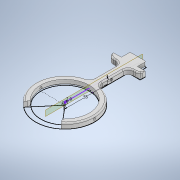
# Autodesk Inventor part: deadbolt enclosure reinforcer from doorknob
Saved by Autodesk Inventor 2022 (Build 260153000, 153)
## iProperties
Created: 2022-04-07
Part Number: deadbolt enclosure reinforcer from doorknob
Material: Generic
Document SubType Name: Modeling
Designer: a-dubs
Density: 1 g/cm^3
Appearance: Default
Author: a-dubs
Autodesk Inventor part; units mm, degrees
ref_plane "YZ Plane" through (0, 0, 0) normal (1, 0, 0) x (0, 1, 0)
ref_plane "XZ Plane" through (0, 0, 0) normal (0, 1, 0) x (-1, 0, 0)
ref_plane "XY Plane" through (0, 0, 0) normal (0, 0, 1) x (1, 0, 0)
sketch "Sketch1" plane through (0, 0, 0) normal (0, 1, 0) x (-1, 0, 0)
  circle A0 centre (0, 0) radius 30.5
  line L0 (0, -30.5) -> (0, -81)
  line L1 (0, -81) -> (0, -92)
  line L2 (0, -92) -> (-10.1, -92)
  line L3 (-10.1, -92) -> (-10.1, -81)
  line L4 (-10.1, -81) -> (0, -81)
  line L5 (-3.0031, -30.5) -> (-3.0031, -30.3518)
  line L6 (-3.0031, -30.5) -> (-3.0031, -81)
  line L7 (-10.1, -81) -> (-10.1, -74.6)
  line L8 (-10.1, -74.6) -> (-3.0031, -74.6)
  line L9 (0, -30.5) -> (0, -36.9)
  circle A1 centre (0, 0) radius 36.9
  line L10 (0, 0) -> (23.7189, 28.267)
  line L11 (0, 0) -> (36.9, 0) construction
  line L12 (0, 0) -> (-23.7189, 28.267)
  line L13 (0, 0) -> (36.9, 0) construction
  line L14 (-10.1, -81) -> (-19.7, -81)
  line L15 (-19.7, -81) -> (-19.7, -74.6)
  line L16 (-19.7, -74.6) -> (-10.1, -74.6)
  line L17 (0, -30.5) -> (-4.8, -30.5)
  line L18 (-4.8, -30.5) -> (-4.8, -30.1199)
  line L19 (-4.8, -30.5) -> (-4.8, -81)
  point P0 (-19.605, 23.3644)
  point P1 (-3.0031, -36.7776)
  point P2 (19.605, 23.3644)
  point P3 (-4.8, -36.5865)
  point P4 (-4.8, -74.6)
  dimension "d0" = 61
  dimension "d1" = 50.5
  dimension "d2" = 11
  dimension "d4" = 10.1
  dimension "d9" = 6.4
  dimension "d10" = 6.4
  dimension "d11" = 50
  dimension "d12" = 130
  dimension "d15" = 9.6
  dimension "d36" = 4.8
  constraints: 40 end point, 6 point on circle, 6 point on line, 5 horizontal, 5 perpendicular, 5 vertical, 2 centre point, 2 coincident, 2 equal length, 1 tangent
  measures "d0" diameter of A0
  measures "d1" distance of L0.start L0.end
  measures "d2" distance of L0.end L1.end
  measures "d4" distance of L1.end L2.end
  measures "d9" distance of L3.end L7.end
  measures "d10" distance of L0.start L9.end
  measures "d11" angle of L11 L10
  measures "d12" angle of L13 L12
  measures "d15" distance of L3.end L14.end
  measures "d36" distance of L0.start L17.end
extrude "Extrusion1" add sketch "Sketch1" along normal blind 6.4 contours L18 L19 A1 L12 A0 | A0 L5 L17 L18 | A0 L17 L5 | L17 L6 A1 L19 | L0 A1 L6 L17 | A1 L6 L8 L19 | L0 L4 L6 A1 | L19 L4 L7 L8 | L8 L6 L4 L19 | L1 L2 L3 L4 | L7 L14 L15 L16
fillet "Fillet1" radius 6.4 1 edges at (4.8, 3.2, -74.6)
chamfer "Chamfer1" distance 3.2 angle 45 1 edges at (19.7, 3.2, -74.6)
fillet "Fillet2" radius 6.4 1 edges at (16.5, 3.2, -74.6)
fillet "Fillet3" radius 6.4 1 edges at (4.8, 3.2, -36.5865)
ref_plane "Work Plane1" through (0, 3.2, -92) normal (-1, 0, 0) x (0, 0, 1)
fillet "Fillet4" radius 1.6 6 edges at (6.1229, 6.4, -37.9299) (36.0247, 6.4, -7.9896) (16.2982, 6.4, -75.0872) (19.0373, 6.4, -77.1373) (6.6745, 6.4, -72.7255) (10.1, 3.2, -92)
mirror "Mirror1" about plane through (0, 3.2, -92) normal (-1, 0, 0) of "Extrusion1", "Fillet3", "Fillet4", "Fillet2", "Chamfer1", "Fillet1"
chamfer "Chamfer2" distance 1.6 angle 45 5 edges at (4.25, 0, -92) (-9.6314, 0, -91.5314) (-10.1, 0, -85.7) (9.6314, 0, -91.5314) (10.1, 0, -85.7)
chamfer "Chamfer3" distance 1.6 angle 45 1 edges at (-28.6606, 0, -10.4316)
fillet "Fillet6" radius 3.2 2 edges at (-19.605, 3.2, 23.3644) (19.605, 3.2, 23.3644)
sketch "Sketch2" plane through (0, 3.2, -92) normal (-1, 0, 0) x (0, 0, 1)
  line L0 (8.7656, 0) -> (93.5, 0)
  line L1 (93.5, 0) -> (38.5, 0)
  circle A0 centre (38.5, 0) radius 1.45
  line L2 (92.05, 0) -> (91.75, 0)
  circle A1 centre (91.75, 0) radius 1.45
  point P0 (92, -3.2)
  dimension "d37" = 55
  dimension "d39" = 2.9
  dimension "d40" = 0.3
  dimension "d41" = 2.9
  constraints: 6 end point, 3 coincident, 3 point on line, 2 centre point, 1 horizontal
  measures "d37" distance of L1.start L1.end
  measures "d39" diameter of A0
  measures "d40" distance of L2.start L2.end
  measures "d41" diameter of A1
extrude "Extrusion2" cut sketch "Sketch2" along normal through all both and the other way through all
body "Solid1"
